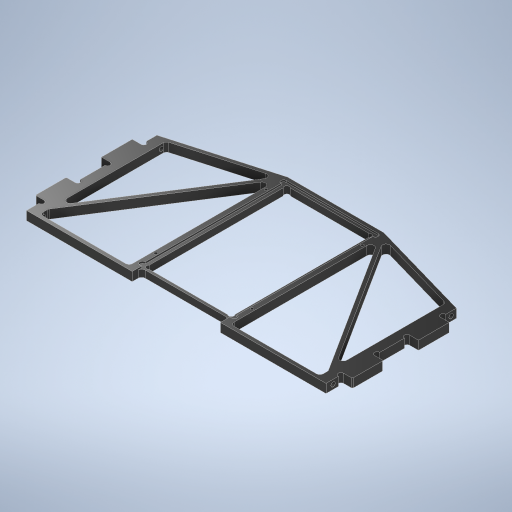
# Autodesk Inventor part: TorsoLowerFrame
Saved by Autodesk Inventor 2024.2 (Build 282272000, 272)
## iProperties
Created: 2024-01-11
Part Number: TorsoLowerFrame
Material: Aluminum 2014-T4
Document SubType Name: Modeling
Designer: Masato Kubotera
Density: 2.8 g/cm^3
Appearance: Glossy - Black
Vendor: meviy
Mass: 47.2837 g
Surface Area: 169.328 cm^2
Volume: 16.887 cm^3
Author: Masato Kubotera
Autodesk Inventor part; units mm, degrees
ref_plane "YZ Plane" through (0, 0, 0) normal (1, 0, 0) x (0, 1, 0)
ref_plane "XZ Plane" through (0, 0, 0) normal (0, 1, 0) x (-1, 0, 0)
ref_plane "XY Plane" through (0, 0, 0) normal (0, 0, 1) x (1, 0, 0)
sketch "Sketch1" plane through (0, 0, 0) normal (0, 0, 1) x (1, 0, 0)
  line L0 (-53, -85) -> (37.5, -85) construction
  line L1 (37.5, 85) -> (-53, 85) construction
  line L2 (0, -85) -> (0, 85) construction
  line L3 (-53, 0) -> (37.5, 0)
  line L4 (10, 90) -> (27.5, 90)
  line L5 (10, 90) -> (10, 85)
  arc A0 (7, 85) -> (10, 85) centre (8.5, 85) ccw
  line L6 (37.5, 85) -> (37.5, -85) construction
  line L7 (-53, -85) -> (-53, 85) construction
  line L8 (31.85, -25.8) -> (-50.75, -25.8) construction
  line L9 (-50.75, -25.8) -> (-50.75, 25.8) construction
  line L10 (-50.75, 25.8) -> (31.85, 25.8) construction
  line L11 (31.85, 25.8) -> (31.85, -25.8) construction
  line L12 (31.85, -25.8) -> (-50.75, 25.8) construction
  line L13 (-50.75, -25.8) -> (31.85, 25.8) construction
  line L14 (32.1, -26.05) -> (-51, -26.05)
  line L15 (-51, -26.05) -> (-51, 26.05)
  line L16 (-51, 26.05) -> (32.1, 26.05)
  line L17 (32.1, 26.05) -> (32.1, -26.05)
  line L18 (32.1, -26.05) -> (-51, 26.05) construction
  line L19 (-51, -26.05) -> (32.1, 26.05) construction
  line L20 (-49.5, 24.3) -> (30.6, 24.3) construction
  line L21 (30.6, 24.3) -> (30.6, -24.3) construction
  line L22 (30.6, -24.3) -> (-49.5, -24.3)
  line L23 (-49.5, -24.3) -> (-49.5, 24.3) construction
  line L24 (-49.5, 24.3) -> (30.6, -24.3) construction
  line L25 (30.6, 24.3) -> (-49.5, -24.3) construction
  line L26 (35.5, 30.8) -> (35.5, 77.5)
  line L27 (30.2417, 79.1864) -> (-43.0052, 32.4864)
  line L28 (-41.93, 28.8) -> (33.5, 28.8)
  line L29 (20.1562, 79.5) -> (-34.4844, 79.5)
  line L30 (37.5, 27.3) -> (-53, 27.3) construction
  arc A1 (33.5, 28.8) -> (35.5, 30.8) centre (33.5, 30.8) ccw
  arc A2 (-43.0052, 32.4864) -> (-41.93, 28.8) centre (-41.93, 30.8) ccw
  arc A3 (21.2314, 75.8136) -> (20.1562, 79.5) centre (20.1562, 77.5) ccw
  arc A4 (32.1, 26.05) -> (29.1, 26.05) centre (30.6, 26.05) ccw
  line L31 (32.1, 25.05) -> (37.5, 25.05)
  arc A5 (30.6, 22.1787) -> (28.4787, 24.3) centre (29.5393, 23.2393) ccw
  arc A6 (-47.3787, 24.3) -> (-49.5, 22.1787) centre (-48.4393, 23.2393) ccw
  arc A7 (-48, 26.05) -> (-51, 26.05) centre (-49.5, 26.05) ccw
  circle A8 centre (21.85, 27.3) radius 1.5 construction
  circle A9 centre (21.85, 27.3) radius 1 construction
  line L32 (-9.45, -25.8) -> (-9.45, 25.7819) construction
  circle A10 centre (-40.75, 27.3) radius 1.5 construction
  circle A11 centre (-40.75, 27.3) radius 1 construction
  circle A12 centre (21.85, 27.3) radius 2.5 construction
  circle A13 centre (-40.75, 27.3) radius 2.5 construction
  line L33 (18.75, 90) -> (18.75, 85) construction
  line L34 (27.5, 90) -> (27.5, 85)
  arc A14 (27.5, 85) -> (30.5, 85) centre (29, 85) ccw
  line L35 (37.5, 85) -> (30.5, 85)
  line L36 (-10, 90) -> (-27.5, 90)
  line L37 (-10, 90) -> (-10, 85)
  arc A15 (-10, 85) -> (-7, 85) centre (-8.5, 85) ccw
  line L38 (-18.75, 90) -> (-18.75, 85) construction
  line L39 (-27.5, 90) -> (-27.5, 85)
  arc A16 (-30.5, 85) -> (-27.5, 85) centre (-29, 85) ccw
  line L40 (7, 85) -> (-7, 85)
  line L41 (33.5, 85) -> (33.5, 79) construction
  line L42 (-33.5, 85) -> (-33.5, 79) construction
  line L43 (-48.5907, 35.445) -> (-36.4073, 78.0499)
  line L44 (-45.5926, 33.2087) -> (21.2314, 75.8136)
  line L45 (-53, 0) -> (-53, 27.3)
  line L46 (-36.5, 85) -> (-30.5, 85)
  arc A17 (-48.5907, 35.445) -> (-45.5926, 33.2087) centre (-46.6678, 34.8951) ccw
  arc A18 (-34.4844, 79.5) -> (-36.4073, 78.0499) centre (-34.4844, 77.5) ccw
  line L47 (30.6, 0) -> (30.6, 22.1787)
  line L48 (28.4787, 24.3) -> (-47.3787, 24.3)
  line L49 (-49.5, 22.1787) -> (-49.5, 0)
  line L50 (37.5, 0) -> (37.5, 85)
  line L51 (-36.5, 85) -> (-53, 27.3)
  line L52 (-53, 27.3) -> (37.5, 85) construction
  line L53 (31.3169, 79.5) -> (33.5, 79.5)
  arc A19 (35.5, 77.5) -> (33.5, 79.5) centre (33.5, 77.5) ccw
  arc A20 (31.3169, 79.5) -> (30.2417, 79.1864) centre (31.3169, 77.5) ccw
  point P0 (0, 0)
  point P1 (50, -85)
  point P2 (-47, 0)
  point P3 (-9.45, 0)
  point P4 (-51, 0)
  point P5 (32.1, 0)
  point P6 (-24.777, 28.8)
  point P7 (35.5, 79.5)
  point P8 (-49.5, 0)
  point P9 (30.6, 0)
  point P10 (32.1, 26.05)
  point P11 (-50.0413, 30.3724)
  point P12 (-35.9926, 79.5)
  point P13 (-49.5, 0)
  point P14 (30.6, 0)
  point P15 (37.5, 25.05)
  point P16 (-53, 27.3)
  point P17 (0, 85)
  dimension "d1" = 170
  dimension "d2" = 1.5
  dimension "d3" = 5
  dimension "d55" = 82.6
  dimension "d56" = 51.6
  dimension "d57" = 0.25
  dimension "d58" = 0.25
  dimension "d62" = 2
  dimension "d66" = 2
  dimension "d71" = 1
  dimension "d81" = 3
  dimension "d82" = 2
  dimension "d85" = 1.5
  dimension "d86" = 1.5
  dimension "d94" = 10
  dimension "d95" = 5
  dimension "d99" = 6
  dimension "d100" = 6
  dimension "d102" = 17.5
  dimension "d103" = 20
  dimension "d104" = 37.5
  dimension "d114" = 2
  dimension "d118" = 5.5
  dimension "d121" = 2
  dimension "d122" = 53
  dimension "d123" = 2
  constraints: 110 end point, 32 point on circle, 31 point on line, 21 centre point, 20 symmetric about line, 18 tangent, 14 midpoint, 10 equal radius, 10 horizontal, 9 parallel, 6 vertical, 5 coincident, 5 collinear, 3 perpendicular, 8 other
  measures "d1" distance of L1.start L0.end
  measures "d2" radius of A0
  measures "d3" distance of L4.start L5.end
  measures "d55" distance of L9.end L10.end
  measures "d56" distance of L8.end L9.end
  measures "d57" distance between parallel lines of L16 L10
  measures "d58" distance between parallel lines of L15 L9
  measures "d62" radius of A1
  measures "d66" distance between parallel lines of L6 L26
  measures "d71" distance of A4.start L31.start
  measures "d81" diameter of A8
  measures "d82" diameter of A9
  measures "d85" distance between parallel lines of L10 L20
  measures "d86" distance between parallel lines of L21 L17
  measures "d94" horizontal distance of L10.end A8.centre
  measures "d95" diameter of A12
  measures "d99" distance of L41.start L41.end
  measures "d100" distance between parallel lines of L34 L41
  measures "d102" distance of L4.start L4.end
  measures "d103" distance between parallel lines of L37 L5
  measures "d104" distance between parallel lines of L6 L2
  measures "d114" distance between parallel lines of L15 L7
  measures "d118" distance between parallel lines of L1 L29
  measures "d121" distance between parallel lines of L43 L51
  measures "d122" distance of point (0, 85) L1.end
  measures "d123" distance between parallel lines of L27 L44
extrude "Extrusion1" add sketch "Sketch1" against normal blind 5 contours L3 L15 L16 L17 L47 A5 L48 A6 L49 | L3 L45 L51 L46 A16 L39 L36 L37 A15 L40 A0 L5 L4 L34 A14 L35 L50 L31 L17 A4 L16 A7 L15 | A7 L16 | L16 A4
extrude "Extrusion2" cut sketch "Sketch1" against normal blind 1 contours L49 A6 L48 A5 L47 L3 | L3 L17 L14 L15 | L3 L15 L16 L17 L47 A5 L48 A6 L49 | A7 L16 | L16 A4
hole "Hole5" at (21.85, 27.3, 0) at (-40.75, 27.3, 0) direction (0, 0, -1) diameter 1.567 end through all thread size "M2x0.4" class "6H" standard "ANSI Metric M Profile"
sketch "Sketch6" plane through (30.5, 85, 0) normal (0, 1, 0) x (1, 0, 0)
  line L0 (0, 5) -> (7, 5) projected
  line L1 (3, 5) -> (3, 0)
  line L2 (7, 0) -> (0, 0) projected
  line L3 (-64, 5) -> (-64, 0)
  line L4 (-67, 5) -> (-61, 5) projected
  point P0 (-30.5, 0)
  point P1 (-86, 5)
  point P2 (-86, 0)
  point P3 (3, 0)
  point P4 (-64, 0)
  point P5 (3, 2.5)
  point P6 (-64, 2.5)
  constraints: 4 end point, 3 midpoint, 2 vertical, 1 point on line
hole "Hole6" at (33.5, 85, -2.5) at (-33.5, 85, -2.5) direction (0, -1, 0) diameter 2.459 depth 10 thread size "M3x0.5" class "6H" standard "ANSI Metric M Profile"
ref_plane "Work Plane1" through (-9.45, 0, -5) normal (1, 0, 0) x (0, 0, -1)
chamfer "Chamfer1" distance 0.5 angle 45 2 edges at (27.5, 90, -2.5) (10, 90, -2.5)
fillet "Fillet1" radius 2 1 edges at (32.1, 25.05, -3)
mirror "Mirror5" about plane through (0, 0, 0) normal (0, 1, 0)
body "Solid1"
